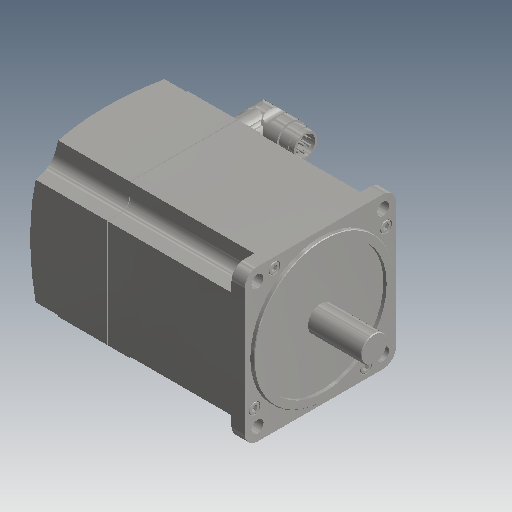
# Autodesk Inventor part: 1574628 EMMS-AS-140-S-HV-RS
Saved by Autodesk Inventor 2021 (Build 250183000, 183)
## iProperties
Part Number: 1574628 EMMS-AS-140-S-HV-RS
Material: Steel AISI 1080
Catalog Web Link: www.cadenas.de
Description: EMMS-AS-servo motor
Vendor: FESTO
Document SubType Name: Modeling
Designer: partserver
Manufacturer: FESTO
Mass: 9600 g
Surface Area: 1690.04 cm^2
Volume: 3761.7 cm^3
Density: 7.85 g/cm^3
Appearance: Steel
Category: PARTsolutions
Company: FESTO
PSOL_IDENT_0: {$CADENAS_DATA\23d-libs\festo\parts\e\emms\emms_as.prj},197 {VTYP=3D},{NB=1574628 EMMS-AS-140-S-HV-R
PSOL_IDENT_1: S},{LINA=1574628 EMMS-AS-140-S-HV-RS},{NN=EMMS-AS},{DATE=30.10.2020 09:47:04},{GEOMDATE=30.10.2020 0
PSOL_IDENT_2: 9:44:16},{VERSION=},{LINEID=5440},{WBVAR=},{WBNUMERIC=}  {NB=1574628 EMMS-AS-140-S-HV-RS},{LINA=1574
PSOL_IDENT_3: 628 EMMS-AS-140-S-HV-RS},{KT=DUMMY},{TNR=1574628},{TYP=EMMS-AS-140-S-HV-RS},{INFO=},{B1=140.500},{B2=
PSOL_IDENT_4: 141.700},{CNSMASSEXACT=9.6000},{VER=9},{VERS=29},{A=209.000},{AA=209},{DP=0},{L=0.0},{L1=0.0},{L2=0.
PSOL_IDENT_5: 0},{L3=0.0},{L4=0.0},{L5=0},{L6=0.0},{L7=0.0},{L8=0.00},{H=0},{H1=0},{H2=0},{D1=0.0},{D2=0.00},{D3=0
PSOL_IDENT_6: .00},{D4=0.0},{D5=0.0},{M=0},{MA=0.000},{M1=0},{M1A=0.000},{EOLDATE=}
NB: 1574628 EMMS-AS-140-S-HV-RS
NN: EMMS-AS
NT: servo motor
NBSYN: $TNR. $TYP.
LINA: 1574628 EMMS-AS-140-S-HV-RS
CATALOG: Festo
TNR: 1574628
TYP: EMMS-AS-140-S-HV-RS
CNSMASSEXACT: 9.6
A: 209
L3: 0
SUPPLIER: FESTO
ARTICLENO: 1574628 EMMS-AS-140-S-HV-RS
BOMINFO: 1574628 EMMS-AS-140-S-HV-RS
CREATOR: CADENAS GmbH
Title: 1574628 EMMS-AS-140-S-HV-RS
Author: Cadenas PARTsolutions
Comments: servo motor
Autodesk Inventor part; units mm, degrees
sketch "Sketch_1" plane through (0, 0, 0) normal (0, 1, 0) x (-1, 0, 0)
  line L0 (41, 250) -> (41, -250)
  arc A0 (-109, 200) -> (-109, -200) centre (41, 0) ccw
  line L1 (-109, -200) -> (-109, 200)
  constraints: 4 end point, 2 point on circle, 1 centre point
revolve "Revolution1" add sketch "Sketch_1" angle 70 mid plane about axis through (-41, 0, 250) along (0, 0, -1)
sketch "Sketch_2" plane through (0, 0, 0) normal (1, 0, 0) x (0, 1, 0)
  line L0 (-72.5, 72.5) -> (-72.5, -72.5)
  line L1 (-72.5, -72.5) -> (72.5, -72.5)
  line L2 (72.5, -72.5) -> (72.5, 72.5)
  line L3 (72.5, 72.5) -> (-72.5, 72.5)
  constraints: 8 end point
extrude "Extrusion1" add sketch "Sketch_2" along normal blind 172.4
sketch "Sketch_9" plane through (12.2, 0, 0) normal (1, 0, 0) x (0, 0, -1)
  line L0 (-255, -255) -> (255, -255)
  line L1 (255, -255) -> (255, 255)
  line L2 (255, 255) -> (-255, 255)
  line L3 (-255, 255) -> (-255, -255)
  line L4 (-70.25, -70.25) -> (70.25, -70.25)
  line L5 (70.25, -70.25) -> (70.25, 70.25)
  line L6 (70.25, 70.25) -> (-70.25, 70.25)
  line L7 (-70.25, 70.25) -> (-70.25, -70.25)
  constraints: 16 end point
extrude "Extrusion2" cut sketch "Sketch_9" along normal blind 196.8
sketch "Sketch_6" plane through (12.2, 0, 0) normal (1, 0, 0) x (0, 0, -1)
  line L0 (-80, -80) -> (80, -80)
  line L1 (80, -80) -> (80, 80)
  line L2 (80, 80) -> (-80, 80)
  line L3 (-80, 80) -> (-80, -80)
  line L4 (-78, -49.25) -> (-58.25, -49.25)
  arc A0 (-49.25, -58.25) -> (-58.25, -49.25) centre (-58.25, -58.25) ccw
  line L5 (-49.25, -58.25) -> (-49.25, -78)
  line L6 (-49.25, -78) -> (49.25, -78)
  line L7 (49.25, -78) -> (49.25, -58.25)
  arc A1 (58.25, -49.25) -> (49.25, -58.25) centre (58.25, -58.25) ccw
  line L8 (58.25, -49.25) -> (78, -49.25)
  line L9 (78, -49.25) -> (78, 49.25)
  line L10 (78, 49.25) -> (58.25, 49.25)
  arc A2 (49.25, 58.25) -> (58.25, 49.25) centre (58.25, 58.25) ccw
  line L11 (49.25, 58.25) -> (49.25, 78)
  line L12 (49.25, 78) -> (-49.25, 78)
  line L13 (-49.25, 78) -> (-49.25, 58.25)
  arc A3 (-58.25, 49.25) -> (-49.25, 58.25) centre (-58.25, 58.25) ccw
  line L14 (-58.25, 49.25) -> (-78, 49.25)
  line L15 (-78, 49.25) -> (-78, -49.25)
  constraints: 32 end point, 8 point on circle, 4 centre point
extrude "Extrusion3" cut sketch "Sketch_6" along normal blind 199.2
sketch "Sketch_3" plane through (0, 0, 0) normal (1, 0, 0) x (0, 1, 0)
  line L0 (-80, 80) -> (-80, -80)
  line L1 (-80, -80) -> (80, -80)
  line L2 (80, -80) -> (80, 80)
  line L3 (80, 80) -> (-80, 80)
  arc A0 (-58.25, 70.25) -> (-70.25, 58.25) centre (-58.25, 58.25) ccw
  line L4 (-70.25, 58.25) -> (-70.25, -58.25)
  arc A1 (-70.25, -58.25) -> (-58.25, -70.25) centre (-58.25, -58.25) ccw
  line L5 (-58.25, -70.25) -> (58.25, -70.25)
  arc A2 (58.25, -70.25) -> (70.25, -58.25) centre (58.25, -58.25) ccw
  line L6 (70.25, -58.25) -> (70.25, 58.25)
  arc A3 (70.25, 58.25) -> (58.25, 70.25) centre (58.25, 58.25) ccw
  line L7 (58.25, 70.25) -> (-58.25, 70.25)
  constraints: 16 end point, 8 point on circle, 4 centre point
extrude "Extrusion4" cut sketch "Sketch_3" along normal blind 12.2
sketch "Sketch_4" plane through (172.7, 0, 0) normal (1, 0, 0) x (0, 0, -1)
  line L0 (-70.85, 49.85) -> (-70.85, -49.85)
  line L1 (-70.85, -49.85) -> (-58.85, -49.85)
  arc A0 (-49.85, -58.85) -> (-58.85, -49.85) centre (-58.85, -58.85) ccw
  line L2 (-49.85, -58.85) -> (-49.85, -70.85)
  line L3 (-49.85, -70.85) -> (49.85, -70.85)
  line L4 (49.85, -70.85) -> (49.85, -58.85)
  arc A1 (58.85, -49.85) -> (49.85, -58.85) centre (58.85, -58.85) ccw
  line L5 (58.85, -49.85) -> (70.85, -49.85)
  line L6 (70.85, -49.85) -> (70.85, 49.85)
  line L7 (70.85, 49.85) -> (58.85, 49.85)
  arc A2 (49.85, 58.85) -> (58.85, 49.85) centre (58.85, 58.85) ccw
  line L8 (49.85, 58.85) -> (49.85, 70.85)
  line L9 (49.85, 70.85) -> (-49.85, 70.85)
  line L10 (-49.85, 70.85) -> (-49.85, 58.85)
  arc A3 (-58.85, 49.85) -> (-49.85, 58.85) centre (-58.85, 58.85) ccw
  line L11 (-58.85, 49.85) -> (-70.85, 49.85)
  constraints: 24 end point, 8 point on circle, 4 centre point
extrude "Extrusion5" add sketch "Sketch_4" against normal blind 45.6
sketch "Sketch7" plane through (12.2, 0, 0) normal (1, 0, 0) x (0, 0, -1)
  point P0 (58.3363, 58.3363)
hole "Hole1" at (12.2, 58.3363, -58.3363) direction (-1, 0, 0) diameter 11.3 depth 12.2
pattern_linear "Rectangular Pattern1" count 2 spacing 116.6726 along (0, 0, 1) count 2 spacing 116.6726 along (0, -1, 0) of "Hole1"
sketch "Sketch_13" plane through (0, 0, 0) normal (0, 0, 1) x (1, 0, 0)
  line L0 (0, 0) -> (-50, 0)
  line L1 (-50, 0) -> (-50, 11.5)
  line L2 (-50, 11.5) -> (-49.5, 12)
  line L3 (-49.5, 12) -> (-0.5, 12)
  line L4 (-0.5, 12) -> (-0.5, 58)
  line L5 (-0.5, 58) -> (-3.5, 58)
  line L6 (-3.5, 58) -> (-3.5, 64.5)
  line L7 (-3.5, 64.5) -> (-3, 65)
  line L8 (-3, 65) -> (0, 65)
  line L9 (0, 65) -> (0, 0)
  line L10 (0, 0) -> (-50, 0)
  constraints: 22 end point
revolve "Revolution2" add sketch "Sketch_13" angle 360 about axis through (0, 0, 0) along (1, 0, 0)
sketch "Sketch_8" plane through (0, 0, -42.5) normal (0, 0, 1) x (1, 0, 0)
  line L0 (6, 61) -> (-1, 61)
  line L1 (-1, 61) -> (-1, 66.5)
  line L2 (-1, 66.5) -> (6, 66.5)
  line L3 (6, 66.5) -> (6, 66)
  line L4 (6, 66) -> (0.6, 66)
  arc A0 (0.6, 66) -> (0, 65.4) centre (0.6, 65.4) ccw
  line L5 (0, 65.4) -> (0, 61)
  line L6 (0, 61) -> (-1, 61)
  constraints: 14 end point, 2 point on circle, 1 centre point
revolve "Revolution3" cut sketch "Sketch_8" angle 360 about axis through (6, 61, -42.5) along (1, 0, 0)
pattern_linear "Rectangular Pattern2" count 2 spacing 105.1404 along (0, -0.1759552, 0.9843982) count 2 spacing 105.1404 along (0, -0.9843982, -0.1759552) of "Revolution3"
sketch "Sketch_18" plane through (0, 0, 0) normal (1, 0, 0) x (0, 1, 0)
  line L0 (59.5566, -40) -> (58.1132, -42.5)
  line L1 (58.1132, -42.5) -> (59.5566, -45)
  line L2 (59.5566, -45) -> (62.4434, -45)
  line L3 (62.4434, -45) -> (63.8868, -42.5)
  line L4 (63.8868, -42.5) -> (62.4434, -40)
  line L5 (62.4434, -40) -> (59.5566, -40)
  constraints: 12 end point
extrude "Extrusion6" cut sketch "Sketch_18" along normal blind 3
pattern_linear "Rectangular Pattern3" count 2 spacing 105.1404 along (0, -0.1759552, 0.9843982) count 2 spacing 105.1404 along (0, -0.9843982, -0.1759552) of "Extrusion6"
sketch "Sketch_11" plane through (0, 42.5, 0) normal (0, 1, 0) x (1, 0, 0)
  line L0 (200.5, -61) -> (180.5, -61)
  line L1 (180.5, -61) -> (180.5, -56.25)
  line L2 (180.5, -56.25) -> (200.5, -56.25)
  line L3 (200.5, -56.25) -> (200.5, -61)
  line L4 (200.5, -61) -> (180.5, -61)
  constraints: 10 end point
revolve "Revolution4" cut sketch "Sketch_11" angle 360 about axis through (200.5, 42.5, 61) along (1, 0, 0)
sketch "Sketch_50" plane through (0, -42.5, 0) normal (0, 1, 0) x (1, 0, 0)
  line L0 (200.5, 61) -> (180.5, 61)
  line L1 (180.5, 61) -> (180.5, 65.75)
  line L2 (180.5, 65.75) -> (200.5, 65.75)
  line L3 (200.5, 65.75) -> (200.5, 61)
  line L4 (200.5, 61) -> (180.5, 61)
  constraints: 10 end point
revolve "Revolution5" cut sketch "Sketch_50" angle 360 about axis through (200.5, -42.5, -61) along (1, 0, 0)
sketch "Sketch_10" plane through (0, 0, -42.5) normal (0, 0, 1) x (1, 0, 0)
  line L0 (200.5, 61) -> (180.5, 61)
  line L1 (180.5, 61) -> (180.5, 65.75)
  line L2 (180.5, 65.75) -> (200.5, 65.75)
  line L3 (200.5, 65.75) -> (200.5, 61)
  line L4 (200.5, 61) -> (180.5, 61)
  constraints: 10 end point
revolve "Revolution6" cut sketch "Sketch_10" angle 360 about axis through (200.5, 61, -42.5) along (1, 0, 0)
sketch "Sketch_51" plane through (0, 0, 42.5) normal (0, 0, 1) x (1, 0, 0)
  line L0 (200.5, -61) -> (180.5, -61)
  line L1 (180.5, -61) -> (180.5, -56.25)
  line L2 (180.5, -56.25) -> (200.5, -56.25)
  line L3 (200.5, -56.25) -> (200.5, -61)
  line L4 (200.5, -61) -> (180.5, -61)
  constraints: 10 end point
revolve "Revolution7" cut sketch "Sketch_51" angle 360 about axis through (200.5, -61, 42.5) along (1, 0, 0)
sketch "Sketch_12" plane through (0, 42.5, 0) normal (0, 1, 0) x (1, 0, 0)
  line L0 (195.5, -61) -> (180.5, -61)
  line L1 (180.5, -61) -> (180.5, -56.75)
  line L2 (180.5, -56.75) -> (195.25, -56.75)
  arc A0 (195.5, -57) -> (195.25, -56.75) centre (195.25, -57) ccw
  line L3 (195.5, -57) -> (195.5, -61)
  line L4 (195.5, -61) -> (180.5, -61)
  constraints: 10 end point, 2 point on circle, 1 centre point
revolve "Revolution8" add sketch "Sketch_12" angle 360 about axis through (195.5, 42.5, 61) along (1, 0, 0)
sketch "Sketch_14" plane through (0, 0, -42.5) normal (0, 0, 1) x (1, 0, 0)
  line L0 (195.5, 61) -> (175.5, 61)
  line L1 (175.5, 61) -> (175.5, 65.25)
  line L2 (175.5, 65.25) -> (195.5, 65.25)
  line L3 (195.5, 65.25) -> (195.5, 61)
  line L4 (195.5, 61) -> (175.5, 61)
  constraints: 10 end point
revolve "Revolution9" add sketch "Sketch_14" angle 360 about axis through (195.5, 61, -42.5) along (1, 0, 0)
sketch "Sketch_54" plane through (0, -42.5, 0) normal (0, 1, 0) x (1, 0, 0)
  line L0 (195.5, 61) -> (175.5, 61)
  line L1 (175.5, 61) -> (175.5, 65.25)
  line L2 (175.5, 65.25) -> (195.5, 65.25)
  line L3 (195.5, 65.25) -> (195.5, 61)
  line L4 (195.5, 61) -> (175.5, 61)
  constraints: 10 end point
revolve "Revolution10" add sketch "Sketch_54" angle 360 about axis through (195.5, -42.5, -61) along (1, 0, 0)
sketch "Sketch_55" plane through (0, 0, 42.5) normal (0, 0, 1) x (1, 0, 0)
  line L0 (195.5, -61) -> (175.5, -61)
  line L1 (175.5, -61) -> (175.5, -56.75)
  line L2 (175.5, -56.75) -> (195.5, -56.75)
  line L3 (195.5, -56.75) -> (195.5, -61)
  line L4 (195.5, -61) -> (175.5, -61)
  constraints: 10 end point
revolve "Revolution11" add sketch "Sketch_55" angle 360 about axis through (195.5, -61, 42.5) along (1, 0, 0)
sketch "Sketch_15" plane through (193.42, 0, 0) normal (1, 0, 0) x (0, 0, -1)
  line L0 (-63, 41.3453) -> (-61, 40.1906)
  line L1 (-61, 40.1906) -> (-59, 41.3453)
  line L2 (-59, 41.3453) -> (-59, 43.6547)
  line L3 (-59, 43.6547) -> (-61, 44.8094)
  line L4 (-61, 44.8094) -> (-63, 43.6547)
  line L5 (-63, 43.6547) -> (-63, 41.3453)
  constraints: 12 end point
extrude "Extrusion7" cut sketch "Sketch_15" along normal blind 12
sketch "Sketch_21" plane through (193.42, 0, 0) normal (1, 0, 0) x (0, 0, -1)
  line L0 (40.5, 59.8453) -> (42.5, 58.6906)
  line L1 (42.5, 58.6906) -> (44.5, 59.8453)
  line L2 (44.5, 59.8453) -> (44.5, 62.1547)
  line L3 (44.5, 62.1547) -> (42.5, 63.3094)
  line L4 (42.5, 63.3094) -> (40.5, 62.1547)
  line L5 (40.5, 62.1547) -> (40.5, 59.8453)
  constraints: 12 end point
extrude "Extrusion8" cut sketch "Sketch_21" along normal blind 12
sketch "Sketch_52" plane through (193.42, 0, 0) normal (1, 0, 0) x (0, 0, -1)
  line L0 (59, -43.6547) -> (61, -44.8094)
  line L1 (61, -44.8094) -> (63, -43.6547)
  line L2 (63, -43.6547) -> (63, -41.3453)
  line L3 (63, -41.3453) -> (61, -40.1906)
  line L4 (61, -40.1906) -> (59, -41.3453)
  line L5 (59, -41.3453) -> (59, -43.6547)
  constraints: 12 end point
extrude "Extrusion9" cut sketch "Sketch_52" along normal blind 12
sketch "Sketch_53" plane through (193.42, 0, 0) normal (1, 0, 0) x (0, 0, -1)
  line L0 (-44.5, -62.1547) -> (-42.5, -63.3094)
  line L1 (-42.5, -63.3094) -> (-40.5, -62.1547)
  line L2 (-40.5, -62.1547) -> (-40.5, -59.8453)
  line L3 (-40.5, -59.8453) -> (-42.5, -58.6906)
  line L4 (-42.5, -58.6906) -> (-44.5, -59.8453)
  line L5 (-44.5, -59.8453) -> (-44.5, -62.1547)
  constraints: 12 end point
extrude "Extrusion10" cut sketch "Sketch_53" along normal blind 12
sketch "Sketch_16" plane through (0, 73.3, 0) normal (0, 1, 0) x (1, 0, 0)
  line L0 (137.9, -22) -> (137.9, -45)
  line L1 (137.9, -45) -> (138.9, -46)
  line L2 (138.9, -46) -> (161.9, -46)
  line L3 (161.9, -46) -> (162.9, -45)
  line L4 (162.9, -45) -> (162.9, -22)
  line L5 (162.9, -22) -> (161.9, -21)
  line L6 (161.9, -21) -> (138.9, -21)
  line L7 (138.9, -21) -> (137.9, -22)
  constraints: 16 end point
extrude "Extrusion11" add sketch "Sketch_16" against normal blind 2.45
sketch "Sketch_20" plane through (140.5, 0, 0) normal (1, 0, 0) x (0, 0, -1)
  line L0 (-23.6, 75.65) -> (-23.6, 73.3)
  line L1 (-23.6, 73.3) -> (-25.85, 73.3)
  line L2 (-25.85, 73.3) -> (-25.85, 75.35)
  line L3 (-25.85, 75.35) -> (-25.55, 75.65)
  line L4 (-25.55, 75.65) -> (-23.6, 75.65)
  line L5 (-23.6, 75.65) -> (-23.6, 73.3)
  constraints: 12 end point
revolve "Revolution12" add sketch "Sketch_20" angle 360 about axis through (140.5, 75.65, 23.6) along (0, 1, 0)
pattern_linear "Rectangular Pattern4" count 2 spacing 19.8 along (1, 0, 0) count 2 spacing 19.8 along (0, 0, 1) of "Revolution12"
sketch "Sketch_23" plane through (0, 0, 33.5) normal (0, 0, 1) x (1, 0, 0)
  line L0 (150.4, 94.2) -> (150.4, 73.3)
  line L1 (150.4, 73.3) -> (143.4, 73.3)
  line L2 (143.4, 73.3) -> (143.4, 82.757)
  line L3 (143.4, 82.757) -> (143.843, 83.2)
  line L4 (143.843, 83.2) -> (145.05, 83.2)
  line L5 (145.05, 83.2) -> (145.05, 84.05)
  line L6 (145.05, 84.05) -> (144.4, 84.7)
  line L7 (144.4, 84.7) -> (144.4, 92.74)
  line L8 (144.4, 92.74) -> (144.86, 93.2)
  line L9 (144.86, 93.2) -> (145.05, 93.2)
  line L10 (145.05, 93.2) -> (145.05, 94.2)
  line L11 (145.05, 94.2) -> (150.4, 94.2)
  line L12 (150.4, 94.2) -> (150.4, 73.3)
  constraints: 26 end point
revolve "Revolution13" add sketch "Sketch_23" angle 360 about axis through (150.4, 94.2, 33.5) along (0, 1, 0)
thread "Thread1" size "M12x1.75" class "6g" standard "ISO Metric profile" full length
sketch "Sketch_24" plane through (0, 75.65, 0) normal (0, 1, 0) x (1, 0, 0)
  line L0 (139.5, -24.1774) -> (140.5, -24.7547)
  line L1 (140.5, -24.7547) -> (141.5, -24.1774)
  line L2 (141.5, -24.1774) -> (141.5, -23.0226)
  line L3 (141.5, -23.0226) -> (140.5, -22.4453)
  line L4 (140.5, -22.4453) -> (139.5, -23.0226)
  line L5 (139.5, -23.0226) -> (139.5, -24.1774)
  constraints: 12 end point
extrude "Extrusion12" cut sketch "Sketch_24" against normal blind 1.1
pattern_linear "Rectangular Pattern5" count 2 spacing 19.8 along (1, 0, 0) count 2 spacing 19.8 along (0, 0, 1) of "Extrusion12"
sketch "Sketch_44" plane through (150.4, 94.2, 33.5) normal (0, 1, 0) x (-1, 0, 0)
  circle A0 centre (0, 0) radius 4.15
  circle A1 centre (2.7433, 0.1918) radius 0.4
  circle A2 centre (1.9445, -1.9445) radius 0.4
  circle A3 centre (1.655, 2.1962) radius 0.4
  circle A4 centre (0, 0) radius 0.4
  circle A5 centre (-0.1918, -2.7433) radius 0.4
  circle A6 centre (-0.5718, 2.6899) radius 0.4
  circle A7 centre (-2.1962, -1.655) radius 0.4
  circle A8 centre (-2.6899, 0.5718) radius 0.4
  constraints: 9 centre point
extrude "Extrusion13" cut sketch "Sketch_44" against normal blind 8.9
sketch "Sketch28" plane through (150.4, 94.2, 33.5) normal (0, 1, 0) x (1, 0, 0)
  point P0 (0, 0)
hole "Hole2" at (150.4, 94.2, 33.5) direction (0, -1, 0) diameter 8.3 depth 1.95
sketch "Sketch_46" plane through (150.4, 94.2, 33.5) normal (0, 1, 0) x (-1, 0, 0)
  line L0 (-3.3279, 2.4794) -> (-2.9274, 2.0789)
  arc A0 (-2.9274, 2.0789) -> (-2.0789, 2.9274) centre (-2.5032, 2.5032) ccw
  line L1 (-2.0789, 2.9274) -> (-2.4794, 3.3279)
  arc A1 (-2.4794, 3.3279) -> (-3.3279, 2.4794) centre (0, 0) ccw
  constraints: 4 end point, 4 point on circle, 2 centre point
extrude "Extrusion14" add sketch "Sketch_46" against normal blind 8.9
sketch "Sketch_47" plane through (150.4, 94.2, 33.5) normal (0, 1, 0) x (-1, 0, 0)
  circle A0 centre (0, 0) radius 4.15
  constraints: 1 centre point
extrude "Extrusion15" cut sketch "Sketch_47" against normal blind 0.5
sketch "Sketch_26" plane through (0, 73.3, 0) normal (0, 1, 0) x (1, 0, 0)
  arc A0 (137.55, 23.15) -> (140.05, 20.65) centre (140.05, 23.15) ccw
  line L0 (140.05, 20.65) -> (160.75, 20.65)
  arc A1 (160.75, 20.65) -> (163.25, 23.15) centre (160.75, 23.15) ccw
  line L1 (163.25, 23.15) -> (163.25, 43.85)
  arc A2 (163.25, 43.85) -> (160.75, 46.35) centre (160.75, 43.85) ccw
  line L2 (160.75, 46.35) -> (140.05, 46.35)
  arc A3 (140.05, 46.35) -> (137.55, 43.85) centre (140.05, 43.85) ccw
  line L3 (137.55, 43.85) -> (137.55, 23.15)
  constraints: 8 end point, 8 point on circle, 4 centre point
extrude "Extrusion16" add sketch "Sketch_26" against normal blind 2.6
sketch "Sketch_30" plane through (140.5, 0, 0) normal (1, 0, 0) x (0, 0, -1)
  line L0 (23.6, 75.6) -> (23.6, 73.25)
  line L1 (23.6, 73.25) -> (21.35, 73.25)
  line L2 (21.35, 73.25) -> (21.35, 75.35)
  line L3 (21.35, 75.35) -> (21.6, 75.6)
  line L4 (21.6, 75.6) -> (23.6, 75.6)
  line L5 (23.6, 75.6) -> (23.6, 73.25)
  constraints: 12 end point
revolve "Revolution14" add sketch "Sketch_30" angle 360 about axis through (140.5, 75.6, -23.6) along (0, 1, 0)
pattern_linear "Rectangular Pattern6" count 2 spacing 19.8 along (1, 0, 0) count 2 spacing 19.8 along (0, 0, -1) of "Revolution14"
sketch "Sketch_31" plane through (0, 75.65, 0) normal (0, 1, 0) x (1, 0, 0)
  line L0 (139.5, 23.0226) -> (140.5, 22.4453)
  line L1 (140.5, 22.4453) -> (141.5, 23.0226)
  line L2 (141.5, 23.0226) -> (141.5, 24.1774)
  line L3 (141.5, 24.1774) -> (140.5, 24.7547)
  line L4 (140.5, 24.7547) -> (139.5, 24.1774)
  line L5 (139.5, 24.1774) -> (139.5, 23.0226)
  constraints: 12 end point
extrude "Extrusion17" cut sketch "Sketch_31" against normal blind 1.1
pattern_linear "Rectangular Pattern7" count 2 spacing 19.8 along (1, 0, 0) count 2 spacing 19.8 along (0, 0, -1) of "Extrusion17"
sketch "Sketch_29" plane through (0, 0, -33.5) normal (0, 0, 1) x (1, 0, 0)
  line L0 (150.4, 100.1) -> (150.4, 73.25)
  line L1 (150.4, 73.25) -> (137.9, 73.25)
  line L2 (137.9, 73.25) -> (137.9, 81.25)
  line L3 (137.9, 81.25) -> (138.4, 81.25)
  line L4 (138.4, 81.25) -> (138.4, 100.1)
  line L5 (138.4, 100.1) -> (150.4, 100.1)
  line L6 (150.4, 100.1) -> (150.4, 73.25)
  constraints: 14 end point
revolve "Revolution15" add sketch "Sketch_29" angle 360 about axis through (150.4, 100.1, -33.5) along (0, 1, 0)
sketch "Sketch_60" plane through (140.5, 0, 0) normal (1, 0, 0) x (0, 0, -1)
  line L0 (23.6, 81.25) -> (23.6, 99.25)
  line L1 (23.6, 99.25) -> (26.6, 99.25)
  line L2 (26.6, 99.25) -> (26.6, 81.25)
  line L3 (26.6, 81.25) -> (23.6, 81.25)
  line L4 (23.6, 81.25) -> (23.6, 99.25)
  constraints: 10 end point
revolve "Revolution16" cut sketch "Sketch_60" angle 360 about axis through (140.5, 81.25, -23.6) along (0, -1, 0)
pattern_linear "Rectangular Pattern8" count 2 spacing 19.8 along (1, 0, 0) count 2 spacing 19.8 along (0, 0, -1) of "Revolution16"
sketch "Sketch_27" plane through (0, 0, -33.5) normal (0, 0, 1) x (1, 0, 0)
  line L0 (163.25, 97.7) -> (111.39, 97.7)
  line L1 (111.39, 97.7) -> (111.39, 108.7)
  line L2 (111.39, 108.7) -> (116.39, 108.7)
  line L3 (116.39, 108.7) -> (116.39, 109.2)
  line L4 (116.39, 109.2) -> (123.39, 109.2)
  line L5 (123.39, 109.2) -> (123.39, 108.7)
  line L6 (123.39, 108.7) -> (125.39, 108.7)
  line L7 (125.39, 108.7) -> (125.39, 110.45)
  line L8 (125.39, 110.45) -> (163.25, 110.45)
  line L9 (163.25, 110.45) -> (163.25, 97.7)
  line L10 (163.25, 97.7) -> (111.39, 97.7)
  constraints: 22 end point
revolve "Revolution17" add sketch "Sketch_27" angle 360 about axis through (163.25, 97.7, -33.5) along (1, 0, 0)
sketch "Sketch_33" plane through (163.25, 0, 0) normal (1, 0, 0) x (0, 0, -1)
  line L0 (28.55, 110.25) -> (28.55, 97.7)
  line L1 (28.55, 97.7) -> (38.45, 97.7)
  line L2 (38.45, 97.7) -> (38.45, 110.25)
  line L3 (38.45, 110.25) -> (28.55, 110.25)
  constraints: 8 end point
extrude "Extrusion18" add sketch "Sketch_33" against normal blind 37.86
sketch "Sketch_36" plane through (163.25, 0, 0) normal (1, 0, 0) x (0, 0, -1)
  line L0 (28.55, 112.25) -> (28.55, 110.25)
  line L1 (28.55, 110.25) -> (38.45, 110.25)
  line L2 (38.45, 110.25) -> (38.45, 112.25)
  line L3 (38.45, 112.25) -> (28.55, 112.25)
  constraints: 8 end point
extrude "Extrusion19" cut sketch "Sketch_36" against normal blind 37.86
sketch "Sketch_34" plane through (0, 110.25, 0) normal (0, 1, 0) x (1, 0, 0)
  arc A0 (139.9, 52.5) -> (144.9, 47.5) centre (139.9, 47.5) ccw
  line L0 (144.9, 47.5) -> (150.5, 46.25)
  arc A1 (150.5, 20.75) -> (150.5, 46.25) centre (150.5, 33.5) ccw
  line L1 (150.5, 20.75) -> (144.9, 19.5)
  arc A2 (144.9, 19.5) -> (139.9, 14.5) centre (139.9, 19.5) ccw
  line L2 (139.9, 14.5) -> (169.9, 14.5)
  line L3 (169.9, 14.5) -> (169.9, 52.5)
  line L4 (169.9, 52.5) -> (139.9, 52.5)
  constraints: 10 end point, 6 point on circle, 3 centre point
extrude "Extrusion20" cut sketch "Sketch_34" against normal blind 27
sketch "Sketch_35" plane through (130.4, 0, 0) normal (1, 0, 0) x (0, 0, -1)
  line L0 (31.6, 110.45) -> (31.6, 110.25)
  line L1 (31.6, 110.25) -> (35.4, 110.25)
  line L2 (35.4, 110.25) -> (35.4, 110.45)
  line L3 (35.4, 110.45) -> (31.6, 110.45)
  constraints: 8 end point
extrude "Extrusion21" add sketch "Sketch_35" along normal blind 3
sketch "Sketch_48" plane through (111.39, 97.7, -33.5) normal (-1, 0, 0) x (0, 1, 0)
  circle A0 centre (0, 0) radius 9
  circle A1 centre (5.1962, 3) radius 0.5
  circle A2 centre (5.1962, -3) radius 1
  circle A3 centre (2.0521, 5.6382) radius 0.5
  circle A4 centre (0, 0) radius 1
  circle A5 centre (0, -6) radius 1
  circle A6 centre (-2.0521, 5.6382) radius 0.5
  circle A7 centre (-5.1962, 3) radius 0.5
  circle A8 centre (-5.1962, -3) radius 1
  constraints: 9 centre point
extrude "Extrusion22" cut sketch "Sketch_48" against normal blind 11.5
sketch "Sketch42" plane through (111.39, 97.7, -33.5) normal (-1, 0, 0) x (0, 0, 1)
  point P0 (0, 0)
hole "Hole3" at (111.39, 97.7, -33.5) direction (1, 0, 0) diameter 18 depth 1
sketch "Sketch_58" plane through (140.5, 0, 0) normal (1, 0, 0) x (0, 0, -1)
  line L0 (23.6, 73.3) -> (23.6, 81.3)
  line L1 (23.6, 81.3) -> (26.1, 81.3)
  line L2 (26.1, 81.3) -> (26.1, 73.3)
  line L3 (26.1, 73.3) -> (25.85, 73.3)
  line L4 (25.85, 73.3) -> (25.85, 75.3525)
  line L5 (25.85, 75.3525) -> (25.6025, 75.6)
  line L6 (25.6025, 75.6) -> (23.6, 75.6)
  line L7 (23.6, 75.6) -> (23.6, 81.3)
  constraints: 16 end point
revolve "Revolution18" cut sketch "Sketch_58" angle 360 about axis through (140.5, 73.3, -23.6) along (0, -1, 0)
pattern_linear "Rectangular Pattern9" count 2 spacing 19.8 along (1, 0, 0) count 2 spacing 19.8 along (0, 0, -1) of "Revolution18"
ref_plane "ANBAU_XY" through (0, 0, 0) normal (1, 0, 0) x (0, 0, -1)
ref_plane "ANBAU_YZ" through (0, 0, 0) normal (0, 0, -1) x (0, 1, 0)
ref_plane "ANBAU_ZX" through (0, 0, 0) normal (0, 1, 0) x (1, 0, 0)
ref_plane "ENCODERLEITUNG_XY" through (150.4, 86.8, 33.5) normal (0, -1, 0) x (-1, 0, 0)
ref_plane "ENCODERLEITUNG_YZ" through (150.4, 86.8, 33.5) normal (-1, 0, 0) x (0, 0, -1)
ref_plane "ENCODERLEITUNG_ZX" through (150.4, 86.8, 33.5) normal (0, 0, -1) x (0, -1, 0)
ref_plane "HGOSCREW_1_XY" through (12.2, 58.3363, -58.3363) normal (-1, 0, 0) x (0, 0, -1)
ref_plane "HGOSCREW_1_YZ" through (12.2, 58.3363, -58.3363) normal (0, 0, -1) x (0, -1, 0)
ref_plane "HGOSCREW_1_ZX" through (12.2, 58.3363, -58.3363) normal (0, -1, 0) x (-1, 0, 0)
ref_plane "HGOSCREW_2_XY" through (12.2, 58.3363, 58.3363) normal (-1, 0, 0) x (0, 0, -1)
ref_plane "HGOSCREW_2_YZ" through (12.2, 58.3363, 58.3363) normal (0, 0, -1) x (0, -1, 0)
ref_plane "HGOSCREW_2_ZX" through (12.2, 58.3363, 58.3363) normal (0, -1, 0) x (-1, 0, 0)
ref_plane "HGOSCREW_3_XY" through (12.2, -58.3363, 58.3363) normal (-1, 0, 0) x (0, 0, -1)
ref_plane "HGOSCREW_3_YZ" through (12.2, -58.3363, 58.3363) normal (0, 0, -1) x (0, -1, 0)
ref_plane "HGOSCREW_3_ZX" through (12.2, -58.3363, 58.3363) normal (0, -1, 0) x (-1, 0, 0)
ref_plane "HGOSCREW_4_XY" through (12.2, -58.3363, -58.3363) normal (-1, 0, 0) x (0, 0, -1)
ref_plane "HGOSCREW_4_YZ" through (12.2, -58.3363, -58.3363) normal (0, 0, -1) x (0, -1, 0)
ref_plane "HGOSCREW_4_ZX" through (12.2, -58.3363, -58.3363) normal (0, -1, 0) x (-1, 0, 0)
ref_plane "MOTORLEITUNG_XY" through (122.89, 97.7, -33.5) normal (1, 0, 0) x (0, 1, 0)
ref_plane "MOTORLEITUNG_YZ" through (122.89, 97.7, -33.5) normal (0, 1, 0) x (0, 0, 1)
ref_plane "MOTORLEITUNG_ZX" through (122.89, 97.7, -33.5) normal (0, 0, 1) x (1, 0, 0)
body "Solid1"
